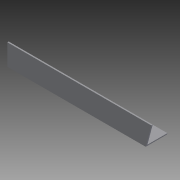
# Autodesk Inventor part: Top Frame Left
Saved by Autodesk Inventor 2015 (Build 190159000, 159)
## iProperties
Created: 2015-01-10
Part Number: Top Frame Left
Material: Generic
Document SubType Name: Modeling
Designer: Chandler Willoughby
Density: 1 g/cm^3
Appearance: Default
Author: Chandler Willoughby
Autodesk Inventor part; units mm, degrees
ref_plane "YZ Plane" through (0, 0, 0) normal (1, 0, 0) x (0, 1, 0)
ref_plane "XZ Plane" through (0, 0, 0) normal (0, 1, 0) x (-1, 0, 0)
ref_plane "XY Plane" through (0, 0, 0) normal (0, 0, 1) x (1, 0, 0)
sketch "Sketch1" plane through (0, 0, 0) normal (1, 0, 0) x (0, 1, 0)
  line L0 (0, 0) -> (50.8, 0)
  line L1 (50.8, 0) -> (50.8, -3.175)
  line L2 (50.8, -3.175) -> (3.175, -3.175)
  line L3 (3.175, -3.175) -> (3.175, -50.8)
  line L4 (3.175, -50.8) -> (0, -50.8)
  line L5 (0, -50.8) -> (0, 0)
  dimension "d1" = 50.8
  dimension "d2" = 3.175
  dimension "d3" = 47.625
  dimension "d4" = 47.625
  dimension "d5" = 3.175
  constraints: 12 end point, 4 perpendicular, 1 horizontal
  measures "d1" distance of L0.start L0.end
  measures "d2" distance of L0.end L1.end
  measures "d3" distance of L1.end L2.end
  measures "d4" distance of L2.end L3.end
  measures "d5" distance of L3.end L4.end
extrude "Extrusion1" add sketch "Sketch1" along normal blind 381
sketch "Sketch2" plane through (0, 0, 0) normal (0, 0, 1) x (1, 0, 0)
  line L0 (381, 0) -> (330.2, 0)
  line L1 (0, 0) -> (381, 0) projected
  line L2 (330.2, 1828.8) -> (812.8, 1828.8)
  line L3 (343.6056, 50.8) -> (330.2, 0)
  line L4 (381, 0) -> (381, 50.8)
  line L5 (381, 50.8) -> (381, 0) projected
  line L6 (381, 50.8) -> (343.6056, 50.8)
  line L7 (0, 50.8) -> (381, 50.8) projected
  dimension "d9" = 50.8
  dimension "d10" = 1828.8
  dimension "d11" = 482.6
  constraints: 10 end point, 2 point on line, 1 collinear
  measures "d9" distance of L0.start L0.end
  measures "d10" distance of L0.end L2.start
  measures "d11" distance of L2.start L2.end
extrude "Extrusion2" cut sketch "Sketch2" against normal blind 381
body "Solid1"
